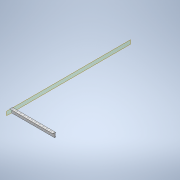
# Autodesk Inventor part: plastic_lip
Saved by Autodesk Inventor 2020 (Build 240168000, 168)
## iProperties
Created: 2020-02-17
Part Number: plastic_lip
Material: Generic
Document SubType Name: Modeling
Designer: erwin
Density: 1 g/cm^3
Appearance: Default
Author: erwin
Autodesk Inventor part; units mm, degrees
ref_plane "YZ Plane" through (0, 0, 0) normal (1, 0, 0) x (0, 1, 0)
ref_plane "XZ Plane" through (0, 0, 0) normal (0, 1, 0) x (-1, 0, 0)
ref_plane "Work Plane1" through (-148, 0, 0) normal (-1, 0, 0) x (0, 0, 1)
sketch "Sketch1" plane through (-148, 0, 0) normal (-1, 0, 0) x (0, 0, 1)
  line L0 (-389.1472, 0) -> (0, 0) projected
  line L1 (-389.1472, 0) -> (-389.1472, -12) projected
  line L2 (0, -12) -> (-389.1472, -12) projected
  line L3 (0, 0) -> (0, -12) projected
  line L4 (1.5, -13.5) -> (-390.6472, -13.5)
  line L5 (-390.6472, -13.5) -> (-390.6472, 1.5)
  line L6 (-390.6472, 1.5) -> (1.5, 1.5)
  line L7 (1.5, 1.5) -> (1.5, -13.5)
  line L8 (-0.5, -13.5) -> (-2, -12)
  line L9 (-3, 0) -> (-1, 2)
  line L10 (-1, 2) -> (3.9889, 2)
  line L11 (3.9889, 2) -> (5.9889, 0)
  line L12 (5.9889, 0) -> (1.5, 0)
  line L13 (3.9889, 2) -> (7.9889, 2)
  line L14 (7.9889, 2) -> (5.9889, 0)
  point P0 (2.9889, 0)
  dimension "d1" = 1.5
  dimension "d2" = 45
  dimension "d3" = 3
  dimension "d4" = 3
  dimension "d5" = 2
  dimension "d6" = 45
  dimension "d7" = 2
  constraints: 22 end point, 4 point on line, 2 horizontal, 2 perpendicular, 1 collinear, 4 other
  measures "d1" distance between parallel lines of L3 L7
  measures "d2" angle of L0 L9
  measures "d3" distance of L0.end L9.start
  measures "d4" distance of L11.end point (2.989, 0)
  measures "d5" distance between parallel lines of L0 L10
  measures "d6" angle of L2 L8
  measures "d7" distance of L2.start L8.end
ref_plane "Work Plane2" through (0, -12, -389.1472) normal (1, 0, 0) x (0, 1, 0)
extrude "Extrusion1" add sketch "Sketch1" against normal up to surface (148 mm away) contours L9 L6 L7 L4 L8 L2 L3 L0 | L9 L10 L11 L12 L7 L6 | L13 L14 L11
equation "\"d4\" = d3"
equation "\"d6\" = d2"
body "Solid1"
